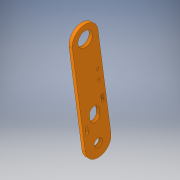
# Autodesk Inventor part: Arm Plates
Saved by Autodesk Inventor 2017 (Build 210142000, 142)
## iProperties
Created: 2017-01-27
Part Number: Arm Plates
Material: Generic
Document SubType Name: Modeling
Designer: Ben
Density: 1 g/cm^3
Appearance: Orange
Author: Ben
Autodesk Inventor part; units mm, degrees
ref_plane "YZ Plane" through (0, 0, 0) normal (1, 0, 0) x (0, 1, 0)
ref_plane "XZ Plane" through (0, 0, 0) normal (0, 1, 0) x (-1, 0, 0)
ref_plane "XY Plane" through (0, 0, 0) normal (0, 0, 1) x (1, 0, 0)
sketch "Sketch1" plane through (0, 0, 0) normal (1, 0, 0) x (0, 1, 0)
  circle A0 centre (0, 0) radius 7.9375
  arc A1 (-3.3867, 25.1732) -> (3.3867, -25.1732) centre (0, 0) ccw
  line L0 (3.3867, -25.1732) -> (192.1857, 0.2268)
  line L1 (0, -25.4) -> (385.0288, -25.4) construction
  circle A2 centre (56.6397, 7.62) radius 31.75 construction
  line L2 (56.6397, 7.62) -> (47.1998, 6.35) construction
  line L3 (57.9097, -1.82) -> (48.4698, -3.09)
  line L4 (45.9298, 15.79) -> (55.3697, 17.06)
  arc A3 (57.9097, -1.82) -> (55.3697, 17.06) centre (56.6397, 7.62) ccw
  arc A4 (45.9298, 15.79) -> (48.4698, -3.09) centre (47.1998, 6.35) ccw
  circle A5 centre (188.7991, 25.4) radius 50.8 construction
  circle A6 centre (188.7991, 25.4) radius 14.2875
  line L5 (137.4291, -7.1399) -> (134.7624, 12.6815) construction
  line L6 (134.7624, 12.6815) -> (95.1195, 7.3482) construction
  line L7 (95.1195, 7.3482) -> (97.7862, -12.4732) construction
  circle A7 centre (47.1998, 6.35) radius 31.75 construction
  line L8 (76.8346, -7.7854) -> (67.3947, -9.0554) construction
  line L9 (76.4926, -5.2429) -> (67.0526, -6.5129)
  line L10 (67.7367, -11.5979) -> (77.1767, -10.3279)
  arc A8 (77.1767, -10.3279) -> (76.4926, -5.2429) centre (76.8346, -7.7854) ccw
  arc A9 (67.0526, -6.5129) -> (67.7367, -11.5979) centre (67.3947, -9.0554) ccw
  line L11 (36.4448, 23.0254) -> (27.0049, 21.7554) construction
  line L12 (36.1028, 25.5679) -> (26.6628, 24.2979)
  line L13 (27.3469, 19.2129) -> (36.7869, 20.4829)
  arc A10 (36.7869, 20.4829) -> (36.1028, 25.5679) centre (36.4448, 23.0254) ccw
  arc A11 (26.6628, 24.2979) -> (27.3469, 19.2129) centre (27.0049, 21.7554) ccw
  line L14 (56.6397, 7.62) -> (76.8346, -7.7854) construction
  line L15 (56.6397, 7.62) -> (36.4448, 23.0254) construction
  line L16 (56.6397, 7.62) -> (88.1062, 11.8533) construction
  circle A12 centre (126.185, 1.4375) radius 2.5527
  circle A13 centre (106.3636, -1.2292) radius 2.5527
  line L17 (126.185, 1.4375) -> (106.3636, -1.2292) construction
  line L18 (126.185, 1.4375) -> (136.0957, 2.7708) construction
  line L19 (106.3636, -1.2292) -> (96.4529, -2.5625) construction
  line L20 (0, 0) -> (239.1455, 32.1733) construction
  arc A14 (192.1857, 0.2268) -> (185.4124, 50.5732) centre (188.7991, 25.4) ccw
  line L21 (185.4124, 50.5732) -> (-3.3867, 25.1732)
  point P0 (51.9197, 6.985)
  point P1 (72.1146, -8.4204)
  point P2 (31.7249, 22.3904)
  dimension "d1" = 63.5
  dimension "d5" = 101.6
  dimension "d0" = 15.875
  dimension "d2" = 50.8
  dimension "d3" = 9.525
  dimension "d4" = 9.525
  dimension "d6" = 28.575
  dimension "d8" = 20
  dimension "d9" = 40
  dimension "d11" = 2.5654
  dimension "d12" = 25.4
  dimension "d15" = 25.4
  dimension "d16" = 45
  dimension "d17" = 47.625
  dimension "d18" = 6.35
  dimension "d19" = 5.1054
  dimension "d20" = 20
  dimension "d21" = 241.3
  constraints: 50 end point, 17 point on circle, 17 tangent, 13 centre point, 10 parallel, 6 midpoint, 5 coincident, 4 equal length, 2 collinear, 2 equal radius, 2 horizontal, 2 perpendicular, 2 point on line, 7 other
  measures "d0" diameter of A0
  measures "d2" diameter of A1
  measures "d3" radius of A3
  measures "d4" distance of L2.start L2.end
  measures "d6" diameter of A6
  measures "d8" distance of L5.start L5.end
  measures "d9" distance of L5.end L6.end
  measures "d11" radius of A9
  measures "d12" distance between parallel lines of L2 L0
  measures "d15" distance of L2.start L8.start
  measures "d16" angle of L2 L14
  measures "d17" distance of point (0, 0) L2.end
  measures "d18" distance from line of L16.end L7
  measures "d19" diameter of A12
  measures "d20" distance of L17.start L17.end
  measures "d21" distance of L20.start L20.end
extrude "Extrusion1" add sketch "Sketch1" along normal blind 6.35
body "Solid1"
